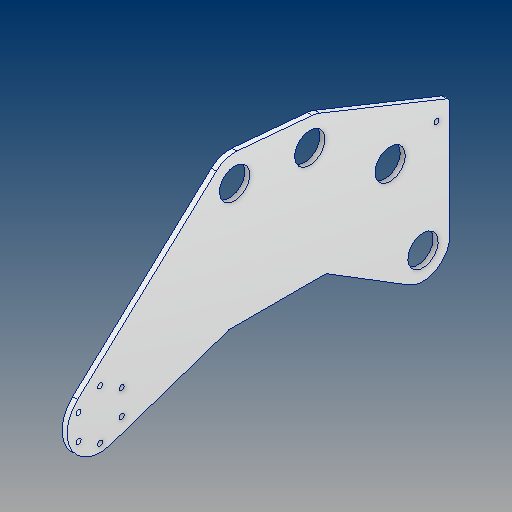
# Autodesk Inventor part: Intake Roller Plate
Saved by Autodesk Inventor 2024.3 (Build 283343000, 343)
## iProperties
Created: 2024-07-25
Part Number: Intake Roller Plate
Material: Aluminum 6061
Document SubType Name: Modeling
Designer: Kenji
Density: 2.7 g/cm^3
Appearance: Aluminum - Flat
Author: Kenji
Autodesk Inventor part; units mm, degrees
ref_plane "YZ Plane" through (0, 0, 0) normal (1, 0, 0) x (0, 1, 0)
ref_plane "XZ Plane" through (0, 0, 0) normal (0, 1, 0) x (-1, 0, 0)
ref_plane "XY Plane" through (0, 0, 0) normal (0, 0, 1) x (1, 0, 0)
sketch "Sketch1" plane through (0, 0, 0) normal (1, 0, 0) x (0, 1, 0)
  line L0 (127, 0) -> (127, -31.75) construction
  line L1 (95.25, -63.5) -> (31.75, -63.5) construction
  line L2 (0, -31.75) -> (0, 0) construction
  arc A0 (95.25, -63.5) -> (127, -31.75) centre (95.25, -31.75) ccw construction
  arc A1 (0, -31.75) -> (31.75, -63.5) centre (31.75, -31.75) ccw construction
  line L3 (0, 0) -> (0, 19.05) construction
  line L4 (0, 19.05) -> (-12.7, 19.05) construction
  line L5 (74.676, 19.05) -> (74.676, 292.1) construction
  circle A2 centre (74.676, 292.1) radius 25.4 construction
  circle A3 centre (74.676, 292.1) radius 31.75 construction
  circle A4 centre (223.901, 292.1) radius 25.4 construction
  circle A5 centre (223.901, 292.1) radius 31.75 construction
  line L6 (-12.7, 19.05) -> (74.676, 19.05) construction
  line L7 (127, 0) -> (0, 0) construction
  line L8 (-12.7, 19.05) -> (-12.7, -285.75) construction
  circle A6 centre (38.1, -114.3) radius 50.8 construction
  circle A7 centre (100.33, -154.8854) radius 25.4 construction
  circle A8 centre (100.33, -154.8854) radius 23.495 construction
  circle A9 centre (100.33, -154.8854) radius 7.62 construction
  circle A10 centre (100.33, -154.8854) radius 14.2875
  circle A11 centre (186.3427, -123.8517) radius 25.4 construction
  circle A12 centre (186.3427, -123.8517) radius 23.495 construction
  circle A13 centre (186.3427, -123.8517) radius 7.62 construction
  circle A14 centre (186.3427, -123.8517) radius 14.2875
  circle A15 centre (237.49, -48.0545) radius 25.4 construction
  circle A16 centre (237.49, -48.0545) radius 23.495 construction
  circle A17 centre (237.49, -48.0545) radius 14.2875
  circle A18 centre (237.49, -48.0545) radius 7.62 construction
  circle A19 centre (177.8, -0.6884) radius 50.8 construction
  line L9 (211.7427, -154.8854) -> (186.3427, -154.8854) construction
  line L10 (186.3427, -154.8854) -> (186.3427, -180.2854) construction
  line L11 (186.3427, -180.2854) -> (211.7427, -180.2854) construction
  line L12 (211.7427, -180.2854) -> (211.7427, -154.8854) construction
  circle A20 centre (199.0427, -167.5854) radius 2.3812
  line L13 (127, 0) -> (127, -63.5) construction
  line L14 (208.5149, -180.2854) -> (100.33, -180.2854)
  line L15 (261.0593, -57.5228) -> (212.9459, -177.2902)
  arc A21 (208.5149, -180.2854) -> (212.9459, -177.2902) centre (208.5149, -175.5102) ccw
  circle A22 centre (243.84, 22.7815) radius 25.4 construction
  circle A23 centre (243.84, 22.7815) radius 23.495 construction
  circle A24 centre (243.84, 22.7815) radius 7.62 construction
  circle A25 centre (243.84, 22.7815) radius 14.2875
  line L16 (262.7886, -50.3223) -> (269.1386, 20.5136)
  arc A26 (261.0593, -57.5228) -> (262.7886, -50.3223) centre (237.49, -48.0545) ccw
  circle A27 centre (118.491, 149.6651) radius 31.115 construction
  circle A28 centre (118.491, 149.6651) radius 7.62 construction
  line L17 (87.376, 149.6651) -> (74.676, 149.6651) construction
  line L18 (74.676, 19.05) -> (127, 19.05) construction
  line L19 (127, 19.05) -> (127, 0) construction
  arc A29 (95.25, -66.04) -> (129.54, -31.75) centre (95.25, -31.75) ccw construction
  line L20 (129.54, -31.75) -> (129.54, 0) construction
  line L21 (141.3154, 170.812) -> (262.4722, 40.0443)
  arc A30 (141.3154, 170.812) -> (89.0204, 139.6839) centre (118.491, 149.6651) ccw
  line L22 (126.7476, 28.2895) -> (89.0204, 139.6839)
  line L23 (126.2857, -64.6546) -> (78.7297, -141.5218)
  arc A31 (78.7297, -141.5218) -> (100.33, -180.2854) centre (100.33, -154.8854) ccw
  line L24 (127, -62.1423) -> (127, 26.7577)
  arc A32 (126.2857, -64.6546) -> (127, -62.1423) centre (122.2248, -62.1423) ccw
  arc A33 (127, 26.7577) -> (126.7476, 28.2895) centre (122.2248, 26.7577) ccw
  arc A34 (269.1386, 20.5136) -> (262.4722, 40.0443) centre (243.84, 22.7815) ccw
  circle A35 centre (118.491, 149.6651) radius 27.94 construction
  circle A36 centre (118.491, 149.6651) radius 23.495 construction
  circle A37 centre (141.986, 149.6651) radius 2.3812
  circle A38 centre (130.2385, 170.0124) radius 2.3812
  circle A39 centre (106.7435, 170.0124) radius 2.3812
  circle A40 centre (94.996, 149.6651) radius 2.3812
  circle A41 centre (106.7435, 129.3178) radius 2.3812
  circle A42 centre (130.2385, 129.3178) radius 2.3812
  point P0 (0, -63.5)
  point P1 (-12.7, -114.3)
  point P2 (211.7427, -167.5854)
  point P3 (211.7427, -123.8517)
  dimension "d58" = 101.6
  dimension "d161" = 46.99
  dimension "d1" = 63.5
  dimension "d2" = 31.75
  dimension "d3" = 19.05
  dimension "d4" = 12.7
  dimension "d7" = 273.05
  dimension "d8" = 50.8
  dimension "d9" = 6.35
  dimension "d10" = 50.8
  dimension "d11" = 6.35
  dimension "d12" = 149.225
  dimension "d13" = 87.376
  dimension "d14" = 127
  dimension "d16" = 304.8
  dimension "d59" = 50.8
  dimension "d60" = 46.99
  dimension "d61" = 15.24
  dimension "d62" = 28.575
  dimension "d70" = 28.575
  dimension "d72" = 129.54
  dimension "d77" = 142.24
  dimension "d78" = 91.44
  dimension "d81" = 101.6
  dimension "d82" = 25.4
  dimension "d83" = 25.4
  dimension "d84" = 4.7625
  dimension "d85" = 12.7
  dimension "d86" = 12.7
  dimension "d88" = 113.03
  dimension "d89" = 91.44
  dimension "d93" = 4.7752
  dimension "d123" = 71.12
  dimension "d124" = 116.84
  dimension "d141" = 62.23
  dimension "d142" = 15.24
  dimension "d143" = 12.7
  dimension "d145" = 2.54
  dimension "d153" = 4.7752
  dimension "d154" = 4.7752
  dimension "d155" = 130.6151
  dimension "d156" = 88.9
  dimension "d160" = 55.88
  dimension "d162" = 4.7625
  dimension "d165" = 360
  constraints: 50 end point, 40 centre point, 30 point on circle, 22 tangent, 16 point on line, 15 coincident, 9 equal radius, 7 horizontal alignment, 6 horizontal, 5 parallel, 5 perpendicular, 3 concentric, 2 collinear, 2 vertical, 1 midpoint, 1 vertical alignment, 24 other
  measures "d1" distance of L0.start point (127, -63.5)
  measures "d2" radius of A0
  measures "d3" distance of L2.end L3.end
  measures "d4" distance of L3.end L4.end
  measures "d7" distance of L5.start L5.end
  measures "d8" diameter of A2
  measures "d9" radial gap between concentric circles of A2 A3
  measures "d10" diameter of A4
  measures "d11" radial gap between concentric circles of A4 A5
  measures "d12" distance of A2.centre A4.centre
  measures "d13" distance of L4.end L5.start
  measures "d14" distance of L0.start L2.end
  measures "d16" distance of L4.end L8.end
  measures "d59" diameter of A7
  measures "d60" diameter of A8
  measures "d61" diameter of A9
  measures "d62" diameter of A10
  measures "d70" diameter of A14
  measures "d72" distance of A12.centre A0.centre
  measures "d77" horizontal distance of A15.centre A0.centre
  measures "d78" distance of point (186.343, -123.852) A16.centre
  measures "d81" diameter of A19
  measures "d82" distance of L11.end L10.end
  measures "d83" distance of L10.end L9.end
  measures "d84" diameter of A20
  measures "d85" distance from line of L9 A20.centre
  measures "d86" distance of point (211.743, -167.585) A20.centre
  measures "d88" distance from line of L8 A7.centre
  measures "d89" distance of A7.centre point (186.343, -123.852)
  measures "d93" radius of A21
  measures "d123" distance of A15.centre A22.centre
  measures "d124" distance from line of L0 A22.centre
  measures "d141" diameter of A27
  measures "d142" diameter of A28
  measures "d143" distance of L17.end L17.start
  measures "d145" radial gap between concentric circles of A0 A29
  measures "d153" radius of A32
  measures "d154" radius of A33
  measures "d155" distance between parallel lines of L18 L17
  measures "d156" distance of L24.start L24.end
  measures "d160" diameter of A35
  measures "d162" diameter of A37
extrude "Extrusion2" add sketch "Sketch1" along normal blind 4.7625 contours L14 A31 L23 A32 L24 A33 L22 A30 L21 A34 L16 A26 L15 A21 | A37 | A38 | A39 | A40 | A41 | A42
extrude "Extrusion3" cut sketch "Sketch1" along normal blind 4.7625 contours A37 | A38 | A39 | A40 | A41 | A42
body "Solid2"
